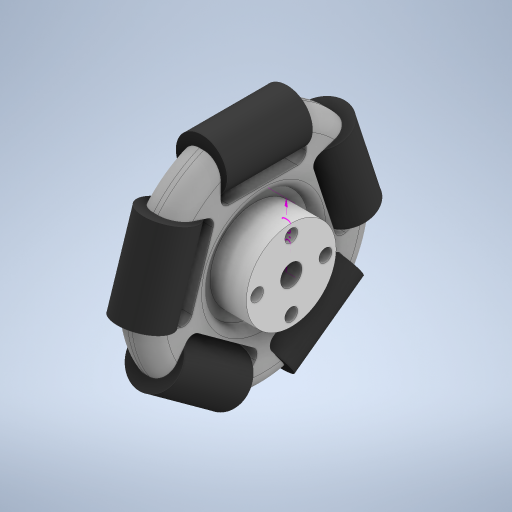
# Autodesk Inventor part: オムニホイール(半分)
Saved by Autodesk Inventor 2024.1 (Build 281209000, 209)
## iProperties
Created: 2024-01-13
Part Number: オムニホイール(半分)
Material: 一般
Document SubType Name: Modeling
Designer: hibik
Density: 1 g/cm^3
Appearance: 既定
Author: hibik
Autodesk Inventor part; units mm, degrees
ref_plane "YZ Plane" through (0, 0, 0) normal (1, 0, 0) x (0, 1, 0)
ref_plane "XZ Plane" through (0, 0, 0) normal (0, 1, 0) x (-1, 0, 0)
ref_plane "XY Plane" through (0, 0, 0) normal (0, 0, 1) x (1, 0, 0)
sketch "スケッチ1" plane through (0, 0, 0) normal (1, 0, 0) x (0, 1, 0)
  circle A0 centre (0, 0) radius 27
  dimension "d0" = 54
  constraints: 1 centre point, 1 coincident
  measures "d0" diameter of A0
extrude "押し出し1" add sketch "スケッチ1" along normal blind 11
extrude "押し出し2" cut sketch "スケッチ1" along normal blind 2
fillet "フィレット1" radius 4 2 edges at (11, -27, 0) (2, -27, 0)
sketch "スケッチ3" plane through (11, 0, 0) normal (1, 0, 0) x (0, 0, -1)
  line L0 (-10, 27) -> (10, 27)
  line L1 (10, 27) -> (10, 17)
  line L2 (8, 15) -> (-8, 15)
  line L3 (-10, 17) -> (-10, 27)
  circle A0 centre (0, 0) radius 27 projected
  line L4 (0, -38.6656) -> (0, 37.9443) projected
  arc A1 (-10, 17) -> (-8, 15) centre (-8, 17) ccw
  arc A2 (8, 15) -> (10, 17) centre (8, 17) ccw
  line L5 (-28.7687, -1.1671) -> (-22.5884, 17.854)
  line L6 (-22.5884, 17.854) -> (-13.0778, 14.7639)
  line L7 (-11.7937, 12.2437) -> (-16.738, -2.9732)
  line L8 (-19.2581, -4.2573) -> (-28.7687, -1.1671)
  arc A3 (-19.2581, -4.2573) -> (-16.738, -2.9732) centre (-18.6401, -2.3552) ccw
  arc A4 (-11.7937, 12.2437) -> (-13.0778, 14.7639) centre (-13.6958, 12.8617) ccw
  line L9 (-7.78, -27.7213) -> (-23.9604, -15.9656)
  line L10 (-23.9604, -15.9656) -> (-18.0825, -7.8754)
  line L11 (-15.2889, -7.433) -> (-2.3446, -16.8375)
  line L12 (-1.9022, -19.6311) -> (-7.78, -27.7213)
  arc A5 (-1.9022, -19.6311) -> (-2.3446, -16.8375) centre (-3.5202, -18.4556) ccw
  arc A6 (-15.2889, -7.433) -> (-18.0825, -7.8754) centre (-16.4645, -9.051) ccw
  line L13 (23.9604, -15.9656) -> (7.78, -27.7213)
  line L14 (7.78, -27.7213) -> (1.9022, -19.6311)
  line L15 (2.3446, -16.8375) -> (15.2889, -7.433)
  line L16 (18.0825, -7.8754) -> (23.9604, -15.9656)
  arc A7 (18.0825, -7.8754) -> (15.2889, -7.433) centre (16.4645, -9.051) ccw
  arc A8 (2.3446, -16.8375) -> (1.9022, -19.6311) centre (3.5202, -18.4556) ccw
  line L17 (22.5884, 17.854) -> (28.7687, -1.1671)
  line L18 (28.7687, -1.1671) -> (19.2581, -4.2573)
  line L19 (16.738, -2.9732) -> (11.7937, 12.2437)
  line L20 (13.0778, 14.7639) -> (22.5884, 17.854)
  arc A9 (13.0778, 14.7639) -> (11.7937, 12.2437) centre (13.6958, 12.8617) ccw
  arc A10 (16.738, -2.9732) -> (19.2581, -4.2573) centre (18.6401, -2.3552) ccw
  point P0 (10, 15)
  point P1 (-10, 15)
  point P2 (0, 27)
  point P3 (-11.1757, 14.1458)
  point P4 (-17.356, -4.8753)
  point P5 (-25.6785, 8.3435)
  point P6 (-16.9069, -6.2574)
  point P7 (-0.7266, -18.0131)
  point P8 (-15.8702, -21.8435)
  point P9 (0.7266, -18.0131)
  point P10 (16.9069, -6.2574)
  point P11 (15.8702, -21.8435)
  point P12 (17.356, -4.8753)
  point P13 (11.1757, 14.1458)
  point P14 (25.6785, 8.3435)
  dimension "d12" = 20
  dimension "d13" = 15
  dimension "d14" = 2
  dimension "d15" = 2
  dimension "d18" = 360
  constraints: 40 end point, 21 point on line, 20 point on circle, 10 centre point, 5 tangent, 2 parallel, 1 horizontal, 1 midpoint, 1 perpendicular, 86 other
  measures "d12" distance of point (10, 15) point (-10, 15)
  measures "d13" distance from line of point (0, 0) L2
  measures "d14" radius of A1
  measures "d15" radius of A2
extrude "押し出し5" cut sketch "スケッチ3" against normal through all contours L0 A0 L3 | L0 L1 A0 | L4 L2 A1 L3 A0 | A0 L1 A2 L2 L4 | L6 A4 L7 A3 L8 A0 | A0 L5 L6 | L20 L17 A0 | A0 L18 A10 L19 A9 L20 | A0 L8 L5 | L17 L18 A0 | L12 L9 A0 | A0 L10 A6 L11 A5 L12 | L14 A8 L15 A7 L16 A0 | A0 L13 L14 | L9 L10 A0 | A0 L16 L13
sketch "スケッチ4" plane through (11, 17, 10) normal (0, 0, -1) x (-1, 0, 0)
  circle A0 centre (4.5, 5) radius 6
  line L0 (4, 8.0799) -> (5, 8.0799) projected
  point P0 (11, -17)
  point P1 (4.5, 8.0799)
  point P2 (0, -2)
  dimension "d22" = 12
  dimension "d23" = 7
  constraints: 1 centre point, 1 midpoint, 1 vertical alignment
  measures "d22" diameter of A0
  measures "d23" vertical distance of A0.centre point (0, -2)
extrude "押し出し6" add sketch "スケッチ4" along normal blind 20
pattern_circular "円形状パターン1" count 5 over 360 about axis through (-10, 0, 0) along (1, 0, 0) of "押し出し6"
sketch "スケッチ6" plane through (11, 0, 0) normal (1, 0, 0) x (0, 0, -1)
  circle A0 centre (0, 0) radius 12.5
  circle A1 centre (0, 0) radius 2.5
  dimension "d35" = 25
  dimension "d36" = 5
  constraints: 3 coincident, 2 centre point
  measures "d35" diameter of A0
  measures "d36" diameter of A1
extrude "押し出し7" add sketch "スケッチ6" against normal blind 11 contours A0 | A1
extrude "押し出し8" cut sketch "スケッチ6" against normal through all contours A1
extrude "押し出し9" cut sketch "スケッチ6" against normal blind 2
fillet "フィレット2" radius 2 1 edges at (11, 0, 12.5)
sketch "スケッチ7" plane through (0, 0, 0) normal (-1, 0, 0) x (0, 0, 1)
  circle A0 centre (0, 0) radius 10.5
  circle A1 centre (0, 0) radius 2.5 projected
  dimension "d45" = 21
  constraints: 1 centre point, 1 coincident
  measures "d45" diameter of A0
extrude "押し出し10" add sketch "スケッチ7" against normal blind 10.5
sketch "スケッチ8" plane through (10.5, 0, 0) normal (1, 0, 0) x (0, 0, -1)
  circle A0 centre (0, 0) radius 10.5
  circle A1 centre (0, 0) radius 2.5 projected
  circle A2 centre (8, 0) radius 2.5
  circle A3 centre (0, 8) radius 2.5
  circle A4 centre (-8, 0) radius 2.5
  circle A5 centre (0, -8) radius 2.5
  circle A6 centre (8, 0) radius 1.5
  circle A7 centre (0, -8) radius 1.5
  circle A8 centre (-8, 0) radius 1.5
  circle A9 centre (0, 8) radius 1.5
  dimension "d48" = 21
  dimension "d49" = 5
  dimension "d52" = 360
  dimension "d54" = 3
  dimension "d55" = 3
  dimension "d56" = 3
  dimension "d57" = 3
  constraints: 9 centre point, 5 coincident, 1 horizontal alignment, 1 tangent, 9 other
  measures "d48" diameter of A0
  measures "d49" diameter of A2
  measures "d54" diameter of A6
  measures "d55" diameter of A7
  measures "d56" diameter of A8
  measures "d57" diameter of A9
extrude "押し出し11" add sketch "スケッチ8" along normal blind 7 contours A3 | A4 | A5 | A0 | A2
